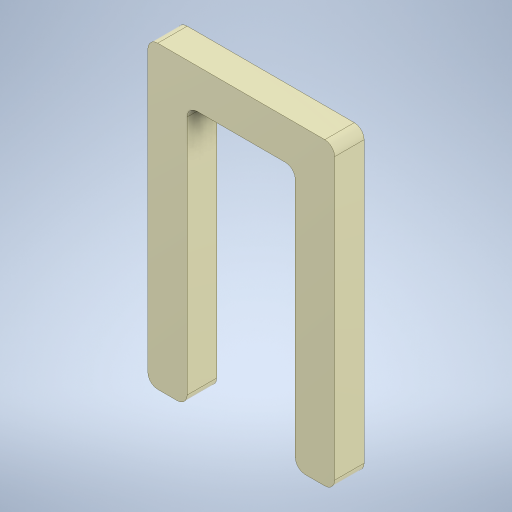
# Autodesk Inventor part: BP_cover
Saved by Autodesk Inventor 2024.3 (Build 283343000, 343)
## iProperties
Created: 2025-11-28
Part Number: BP_cover
Material: 一般
Document SubType Name: Modeling
Designer: 佐藤智貴
Density: 1 g/cm^3
Appearance: 滑らか - 灰色
Author: 佐藤智貴
Autodesk Inventor part; units mm, degrees
ref_plane "YZ Plane" through (0, 0, 0) normal (1, 0, 0) x (0, 1, 0)
ref_plane "XZ Plane" through (0, 0, 0) normal (0, 1, 0) x (-1, 0, 0)
ref_plane "XY Plane" through (0, 0, 0) normal (0, 0, 1) x (1, 0, 0)
sketch "スケッチ1" plane through (0, 0, 0) normal (0, 0, 1) x (1, 0, 0)
  line L0 (0, 0) -> (190, 0)
  line L1 (190, 0) -> (190, 305)
  line L2 (190, 305) -> (0, 305)
  line L3 (0, 305) -> (0, 0)
  line L4 (0, 305) -> (40, 305)
  line L5 (40, 305) -> (40, 0)
  line L6 (40, 0) -> (0, 0)
  line L7 (0, 0) -> (0, 305)
  line L8 (190, 0) -> (150, 0)
  line L9 (150, 0) -> (150, 305)
  line L10 (150, 305) -> (190, 305)
  line L11 (190, 305) -> (190, 0)
  line L12 (0, 305) -> (190, 305)
  line L13 (190, 305) -> (190, 265)
  line L14 (190, 265) -> (0, 265)
  line L15 (0, 265) -> (0, 305)
  point P0 (40, 265)
  point P1 (150, 265)
  dimension "d0" = 305
  dimension "d1" = 190
  dimension "d2" = 40
  dimension "d3" = 40
  dimension "d4" = 40
  constraints: 32 end point, 8 parallel, 4 horizontal, 4 perpendicular, 3 point on line
  measures "d0" distance of L0.end L1.end
  measures "d1" distance of L1.end L2.end
  measures "d2" distance between parallel lines of L2 L14
  measures "d3" distance between parallel lines of L3 L5
  measures "d4" distance between parallel lines of L1 L9
extrude "押し出し1" add sketch "スケッチ1" along normal blind 30 contours L3 L14 L5 L0 | L3 L2 L5 L14 | L9 L14 L1 L0 | L5 L2 L9 L14 | L9 L2 L1 L14
fillet "フィレット1" radius 10 8 edges at (0, 305, 15) (0, 0, 15) (190, 305, 15) (40, 265, 15) (150, 265, 15) (150, 0, 15) (190, 0, 15) (40, 0, 15)
equation "\"d3\" = d2"
equation "\"d4\" = d2"
